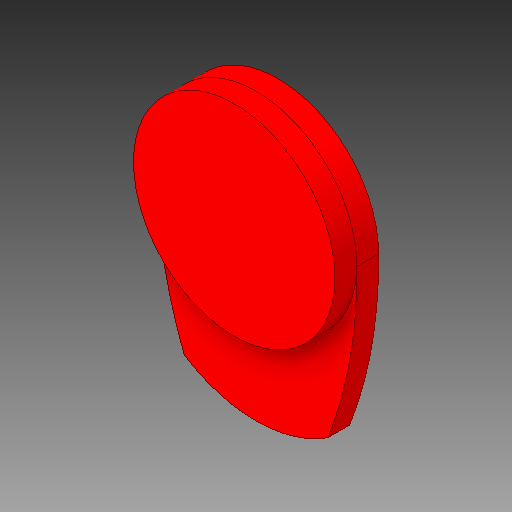
# Autodesk Inventor part: brazocuadrado
Saved by Autodesk Inventor 2019 (Build 230136000, 136)
## iProperties
Part Number: brazocuadrado
Material: Genérico
Document SubType Name: Chapa
Designer: Kevin
Density: 1 g/cm^3
Sheet Metal Rule: Por defecto_mm
Appearance: Valor por defecto
Author: Kevin
Autodesk Inventor part; units mm, degrees
ref_plane "Plano de trabajo5" through (38.9749, 57.0341, 41) normal (0, 0, 1) x (1, 0, 0)
sketch "Boceto10" plane through (38.9749, 57.0341, 41) normal (0, 0, 1) x (1, 0, 0)
  arc A0 (9.2555, -0.0835) -> (-9.2551, 0.0106) centre (0.0004, 0) ccw
  arc A1 (-9.2551, 0.0106) -> (-6.6027, -15.0198) centre (30.7389, -0.6809) ccw
  arc A2 (6.605, -15.0198) -> (9.2555, -0.0835) centre (-30.7399, -0.6895) ccw
  arc A3 (-6.6027, -15.0198) -> (6.605, -15.0198) centre (0.0012, -4.9335) ccw
  constraints: 8 point on circle, 4 centre point
extrude "Extrusión7" add sketch "Boceto10" along normal blind 2
ref_plane "Plano de trabajo4" through (38.9749, 57.0341, -1) normal (0, 0, -1) x (-1, 0, 0)
ref_plane "Plano de trabajo2" through (0, 0, 0) normal (0, 0, 1) x (1, 0, 0)
sketch "Boceto34" plane through (38.9749, 57.0341, 43) normal (0, 0, 1) x (1, 0, 0)
  circle A0 centre (0, 0) radius 9.2555
  point P0 (-38.9749, -57.0341)
  constraints: 1 centre point
extrude "Extrusión26" add sketch "Boceto34" along normal blind 2
equation "\"Radio_pliegue\" = Grosor"
equation "\"Anchura_desahogo_plegado\" = Grosor"
equation "\"Profundidad_desahogo_plegado\" = 0.5 * Grosor"
equation "\"Tamaño_destalonado\" = 4 * Grosor"
equation "\"Remanente_mínimo\" = 2 * Grosor"
equation "\"Radiodetransición\" = Radio_pliegue"
equation "\"Tamaño_de_radio_de_Jacobi\" = Radio_pliegue"
equation "\"TamañoSeparación\" = Grosor"
equation "\"Grosor\" = 0.5"
